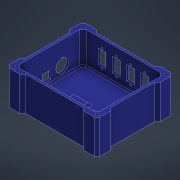
# Autodesk Inventor part: Case
Saved by Autodesk Inventor 2021.3 (Build 253353000, 353)
## iProperties
Created: 2020-02-03
Part Number: Case
Material: Generic
Document SubType Name: Modeling
Designer: Alex
Density: 1 g/cm^3
Appearance: Default
Author: Alex
Autodesk Inventor part; units mm, degrees
ref_plane "YZ Plane" through (0, 0, 0) normal (1, 0, 0) x (0, 1, 0)
ref_plane "XZ Plane" through (0, 0, 0) normal (0, 1, 0) x (-1, 0, 0)
ref_plane "XY Plane" through (0, 0, 0) normal (0, 0, 1) x (1, 0, 0)
sketch "Sketch1" plane through (0, 0, 0) normal (0, 1, 0) x (-1, 0, 0)
  line L0 (-60, 50) -> (-41, 50) construction
  line L1 (60, 50) -> (60, 31) construction
  line L2 (60, -50) -> (41, -50) construction
  line L3 (-60, -50) -> (-60, -31) construction
  line L4 (-60, 50) -> (60, -50) construction
  line L5 (60, 50) -> (-60, -50) construction
  line L6 (41, -50) -> (45, -54)
  line L7 (45, -54) -> (60, -54)
  line L8 (60, -54) -> (64, -50)
  line L9 (64, -50) -> (64, -35)
  line L10 (64, -35) -> (60, -31)
  line L11 (-41, -50) -> (-45, -54)
  line L12 (-45, -54) -> (-60, -54)
  line L13 (-60, -54) -> (-64, -50)
  line L14 (-64, -50) -> (-64, -35)
  line L15 (-64, -35) -> (-60, -31)
  line L16 (-60, 31) -> (-64, 35)
  line L17 (-64, 35) -> (-64, 50)
  line L18 (-64, 50) -> (-60, 54)
  line L19 (-60, 54) -> (-45, 54)
  line L20 (-45, 54) -> (-41, 50)
  line L21 (41, 50) -> (45, 54)
  line L22 (45, 54) -> (60, 54)
  line L23 (60, 54) -> (64, 50)
  line L24 (64, 50) -> (64, 35)
  line L25 (64, 35) -> (60, 31)
  line L26 (41, -50) -> (-41, -50)
  line L27 (60, -31) -> (60, -50) construction
  line L28 (60, 31) -> (60, -31)
  line L29 (41, 50) -> (60, 50) construction
  line L30 (-41, 50) -> (41, 50)
  line L31 (-60, 31) -> (-60, 50) construction
  line L32 (-41, -50) -> (-60, -50) construction
  line L33 (-60, -31) -> (-60, 31)
  point P0 (0, 0)
  point P1 (0, 0)
  point P2 (0, 0)
  dimension "d4" = 120
  dimension "d5" = 100
  dimension "d6" = 45
  dimension "d7" = 15
  dimension "d8" = 4
  dimension "d9" = 4
  dimension "d12" = 45
  dimension "d13" = 4
  constraints: 68 end point, 21 parallel, 16 perpendicular, 7 equal length, 6 collinear, 6 vertical alignment, 5 horizontal, 3 horizontal alignment, 3 midpoint, 1 coincident, 1 point on line
  measures "d4" distance of L2.start L3.start
  measures "d5" distance of L1.start L2.start
  measures "d6" angle of L6 L2
  measures "d7" distance of L6.end L7.end
  measures "d8" distance between parallel lines of L7 L2
  measures "d9" horizontal distance of L7.end L8.end
  measures "d12" angle of L2 L11
  measures "d13" distance between parallel lines of L14 L3
extrude "Extrusion2" add sketch "Sketch1" along normal blind 3
sketch "Sketch2" plane through (0, 3, 0) normal (0, 1, 0) x (1, 0, 0)
  line L0 (-64, 50) -> (-64, 35) projected
  line L1 (-64, 35) -> (-60, 31) projected
  line L2 (-60, 31) -> (-60, -31) projected
  line L3 (-60, -31) -> (-64, -35) projected
  line L4 (-64, -35) -> (-64, -50) projected
  line L5 (-64, -50) -> (-60, -54) projected
  line L6 (-60, -54) -> (-45, -54) projected
  line L7 (-45, -54) -> (-41, -50) projected
  line L8 (-41, -50) -> (41, -50) projected
  line L9 (41, -50) -> (45, -54) projected
  line L10 (45, -54) -> (60, -54) projected
  line L11 (60, -54) -> (64, -50) projected
  line L12 (64, -50) -> (64, -35) projected
  line L13 (64, -35) -> (60, -31) projected
  line L14 (60, -31) -> (60, 31) projected
  line L15 (60, 31) -> (64, 35) projected
  line L16 (64, 35) -> (64, 50) projected
  line L17 (64, 50) -> (60, 54) projected
  line L18 (60, 54) -> (45, 54) projected
  line L19 (45, 54) -> (41, 50) projected
  line L20 (41, 50) -> (-41, 50) projected
  line L21 (-41, 50) -> (-45, 54) projected
  line L22 (-45, 54) -> (-60, 54) projected
  line L23 (-60, 54) -> (-64, 50) projected
  line L24 (-42.2426, 47) -> (42.2426, 47)
  line L25 (42.2426, 47) -> (46.2426, 51) construction
  line L26 (46.2426, 51) -> (58.7574, 51) construction
  line L27 (58.7574, 51) -> (61, 48.7574) construction
  line L28 (61, 48.7574) -> (61, 36.2426) construction
  line L29 (61, 36.2426) -> (57, 32.2426) construction
  line L30 (57, 32.2426) -> (57, -32.2426)
  line L31 (57, -32.2426) -> (61, -36.2426) construction
  line L32 (61, -36.2426) -> (61, -48.7574) construction
  line L33 (61, -48.7574) -> (58.7574, -51) construction
  line L34 (58.7574, -51) -> (46.2426, -51) construction
  line L35 (46.2426, -51) -> (42.2426, -47) construction
  line L36 (42.2426, -47) -> (-42.2426, -47)
  line L37 (-42.2426, -47) -> (-46.2426, -51) construction
  line L38 (-46.2426, -51) -> (-58.7574, -51) construction
  line L39 (-58.7574, -51) -> (-61, -48.7574) construction
  line L40 (-61, -48.7574) -> (-61, -36.2426) construction
  line L41 (-61, -36.2426) -> (-57, -32.2426) construction
  line L42 (-57, -32.2426) -> (-57, 32.2426)
  line L43 (-57, 32.2426) -> (-61, 36.2426) construction
  line L44 (-61, 36.2426) -> (-61, 48.7574) construction
  line L45 (-61, 48.7574) -> (-58.7574, 51) construction
  line L46 (-58.7574, 51) -> (-46.2426, 51) construction
  line L47 (-46.2426, 51) -> (-42.2426, 47) construction
  line L48 (-42.2426, 47) -> (-52.2426, 47)
  line L49 (-52.2426, 47) -> (-57, 42.2426)
  line L50 (-57, 42.2426) -> (-57, 32.2426)
  line L51 (-57, -32.2426) -> (-57, -42.2426)
  line L52 (-57, -42.2426) -> (-52.2426, -47)
  line L53 (-52.2426, -47) -> (-42.2426, -47)
  line L54 (42.2426, -47) -> (52.2426, -47)
  line L55 (52.2426, -47) -> (57, -42.2426)
  line L56 (57, -42.2426) -> (57, -32.2426)
  line L57 (57, 32.2426) -> (57, 42.2426)
  line L58 (57, 42.2426) -> (52.2426, 47)
  line L59 (52.2426, 47) -> (42.2426, 47)
  point P0 (0, 0)
  dimension "d16" = 3
  dimension "d17" = 10
  constraints: 72 end point, 7 equal length, 4 perpendicular, 2 point on line, 1 horizontal, 1 vertical, 23 other
  measures "d16" distance between parallel lines of L20 L24
  measures "d17" distance of L24.start L48.end
extrude "Extrusion3" add sketch "Sketch2" along normal blind 45
sketch "Sketch4" plane through (0, 3, 0) normal (0, 1, 0) x (1, 0, 0)
  line L0 (45, 54) -> (41, 50) construction
  line L1 (41, 50) -> (-41, 50) construction
  line L2 (-41, 50) -> (-45, 54) construction
  line L3 (-45, 54) -> (-60, 54) construction
  line L4 (-60, 54) -> (-64, 50) construction
  line L5 (-64, 50) -> (-64, 35) construction
  line L6 (-64, 35) -> (-60, 31) construction
  line L7 (-60, 31) -> (-60, -31) construction
  line L8 (-60, -31) -> (-64, -35) construction
  line L9 (-64, -35) -> (-64, -50) construction
  line L10 (-64, -50) -> (-60, -54) construction
  line L11 (-60, -54) -> (-45, -54) construction
  line L12 (-45, -54) -> (-41, -50) construction
  line L13 (-41, -50) -> (41, -50) construction
  line L14 (41, -50) -> (45, -54) construction
  line L15 (45, -54) -> (60, -54) construction
  line L16 (60, -54) -> (64, -50) construction
  line L17 (64, -50) -> (64, -35) construction
  line L18 (64, -35) -> (60, -31) construction
  line L19 (60, -31) -> (60, 31) construction
  line L20 (60, 31) -> (64, 35) construction
  line L21 (64, 35) -> (64, 50) construction
  line L22 (64, 50) -> (60, 54) construction
  line L23 (60, 54) -> (45, 54) construction
  line L24 (-52.2426, 47) -> (52.2426, 47) construction
  line L25 (52.2426, 47) -> (57, 42.2426) construction
  line L26 (57, 42.2426) -> (57, -42.2426) construction
  line L27 (57, -42.2426) -> (52.2426, -47) construction
  line L28 (52.2426, -47) -> (-52.2426, -47) construction
  line L29 (-52.2426, -47) -> (-57, -42.2426) construction
  line L30 (-57, -42.2426) -> (-57, 42.2426) construction
  line L31 (-57, 42.2426) -> (-52.2426, 47) construction
  line L32 (-52.2426, 47) -> (-57, 42.2426) construction
  line L33 (-57, 42.2426) -> (-57, -42.2426) construction
  line L34 (-57, -42.2426) -> (-52.2426, -47) construction
  line L35 (-52.2426, -47) -> (52.2426, -47) construction
  line L36 (52.2426, -47) -> (57, -42.2426) construction
  line L37 (57, -42.2426) -> (57, 42.2426) construction
  line L38 (57, 42.2426) -> (52.2426, 47) construction
  line L39 (52.2426, 47) -> (-52.2426, 47) construction
  line L40 (-54, 11.34) -> (47.6, 11.34) construction
  line L41 (47.6, 11.34) -> (47.6, -42) construction
  line L42 (47.6, -42) -> (-54, -42) construction
  line L43 (-54, -42) -> (-54, 11.34) construction
  line L44 (9.6, -4) -> (14.6, -4)
  line L45 (14.6, -4) -> (14.6, -9)
  line L46 (14.6, -9) -> (9.6, -9)
  line L47 (9.6, -9) -> (9.6, -4)
  line L48 (9.6, -4) -> (14.6, -9) construction
  line L49 (14.6, -4) -> (9.6, -9) construction
  line L50 (45.02, -42) -> (40.02, -42)
  line L51 (40.02, -42) -> (40.02, -37)
  line L52 (40.02, -37) -> (45.02, -37)
  line L53 (45.02, -37) -> (45.02, -42)
  line L54 (45.02, -42) -> (40.02, -37) construction
  line L55 (40.02, -42) -> (45.02, -37) construction
  line L56 (-24, 1.34) -> (-4, 1.34)
  line L57 (-4, 1.34) -> (-4, -32)
  line L58 (-4, -32) -> (-24, -32)
  line L59 (-24, -32) -> (-24, 1.34)
  line L60 (21, 1.34) -> (31, 1.34)
  line L61 (31, 1.34) -> (31, -32)
  line L62 (31, -32) -> (21, -32)
  line L63 (21, -32) -> (21, 1.34)
  point P0 (-40, -39.5)
  point P1 (-38.7, 8.7)
  point P2 (12.1, -34.4)
  point P3 (12.1, -6.5)
  point P4 (36.2, 8.7)
  point P5 (42.52, -39.5)
  dimension "d20" = 53.34
  dimension "d21" = 101.6
  dimension "d23" = 5
  dimension "d24" = 3
  dimension "d25" = 14
  dimension "d26" = 1.3
  dimension "d27" = 50.8
  dimension "d29" = 2.5
  dimension "d30" = 5.1
  dimension "d31" = 27.9
  dimension "d32" = 15.2
  dimension "d33" = 24.1
  dimension "d34" = 96.52
  dimension "d35" = 30
  dimension "d36" = 50
  dimension "d37" = 10
  dimension "d38" = 10
  dimension "d39" = 75
  dimension "d40" = 85
  dimension "d41" = 5
  constraints: 48 end point, 10 parallel, 5 horizontal, 5 perpendicular, 4 midpoint, 3 equal length, 2 collinear, 2 horizontal alignment, 1 vertical alignment
  measures "d20" distance of L40.end L41.end
  measures "d21" distance of L40.start L40.end
  measures "d23" distance between parallel lines of L42 L28
  measures "d24" distance between parallel lines of L30 L43
  measures "d25" distance from line of point (-40, -39.5) L43
  measures "d26" horizontal distance of point (-38.7, 8.7) point (-40, -39.5)
  measures "d27" horizontal distance of point (12.1, -6.5) point (-38.7, 8.7)
  measures "d29" distance from line of point (42.52, -39.5) L42
  measures "d30" vertical distance of point (12.1, -34.4) point (-40, -39.5)
  measures "d31" distance of point (12.1, -6.5) point (12.1, -34.4)
  measures "d32" vertical distance of point (36.2, 8.7) point (12.1, -6.5)
  measures "d33" horizontal distance of point (36.2, 8.7) point (12.1, -6.5)
  measures "d34" distance from line of point (42.52, -39.5) L43
  measures "d35" distance between parallel lines of L59 L43
  measures "d36" distance between parallel lines of L57 L43
  measures "d37" distance between parallel lines of L56 L40
  measures "d38" distance between parallel lines of L58 L42
  measures "d39" distance between parallel lines of L63 L43
  measures "d40" distance between parallel lines of L61 L43
  measures "d41" distance of L45.end L46.end
extrude "Extrusion4" add sketch "Sketch4" along normal blind 3
chamfer "Chamfer1" distance 3 angle 45 16 edges at (-14, 3, 32) (-4, 3, 15.33) (21, 3, 15.33) (-24, 3, 15.33) (26, 3, 32) (40.02, 3, 39.5) (42.52, 3, 37) (45.02, 3, 39.5) (42.52, 3, 42) (9.6, 3, 6.5) (12.1, 3, 9) (14.6, 3, 6.5) (12.1, 3, 4) (26, 3, -1.34) (-14, 3, -1.34) (31, 3, 15.33)
sketch "Sketch5" plane through (0, 6, 0) normal (0, 1, 0) x (1, 0, 0)
  line L0 (14.6, -9) -> (14.6, -4) construction
  line L1 (14.6, -4) -> (9.6, -4) construction
  line L2 (9.6, -4) -> (9.6, -9) construction
  line L3 (9.6, -9) -> (14.6, -9) construction
  line L4 (40.02, -42) -> (45.02, -42) construction
  line L5 (45.02, -42) -> (45.02, -37) construction
  line L6 (45.02, -37) -> (40.02, -37) construction
  line L7 (40.02, -37) -> (40.02, -42) construction
  point P0 (0, 0)
  point P1 (12.1, -6.5)
  point P2 (42.52, -39.5)
  point P3 (14.6, -6.5)
  point P4 (45.02, -39.5)
  point P5 (12.1, -4)
  point P6 (42.52, -37)
  constraints: 4 midpoint, 2 horizontal alignment, 2 vertical alignment
hole "Hole1" at (12.1, 6, 6.5) at (42.52, 6, 39.5) direction (0, -1, 0) diameter 4 depth 5
sketch "Sketch6" plane through (-57, 3, 42.2426) normal (1, 0, 0) x (0, 0, -1)
  line L0 (46.5826, 0) -> (7.2426, 0) construction
  line L1 (7.2426, 0) -> (46.5826, 0) construction
  line L2 (7.2426, 0) -> (46.5826, 0) construction
  line L3 (46.5826, 0) -> (7.2426, 0) construction
  line L4 (-2.7574, 0) -> (8.2426, 0) construction
  line L5 (-4.7574, 0) -> (0, 0) construction
  line L6 (0, 0) -> (84.4853, 0) construction
  line L7 (84.4853, 0) -> (89.2426, 0) construction
  line L8 (89.2426, 0) -> (84.4853, 0) construction
  line L9 (84.4853, 0) -> (0, 0) construction
  line L10 (0, 0) -> (-4.7574, 0) construction
  line L11 (8.2426, 0) -> (-2.7574, 0) construction
  line L12 (41.2426, 0) -> (30.2426, 0) construction
  line L13 (30.2426, 0) -> (41.2426, 0) construction
  line L14 (0.2426, 0) -> (53.5826, 0) construction
  line L15 (43.5826, 3) -> (10.2426, 3) construction
  line L16 (10.2426, 3) -> (43.5826, 3) construction
  line L17 (43.5826, 3) -> (46.5826, 0) construction
  line L18 (46.5826, 0) -> (43.5826, 3) construction
  line L19 (10.2426, 3) -> (7.2426, 0) construction
  line L20 (10.2426, 3) -> (7.2426, 0) construction
  line L21 (84.4853, 0) -> (0, 0) construction
  line L22 (84.4853, 0) -> (84.4853, 45) construction
  line L23 (0, 45) -> (84.4853, 45) construction
  line L24 (0, 0) -> (0, 45) construction
  line L25 (31.8326, 16.2) -> (44.3326, 16.2)
  line L26 (44.3326, 16.2) -> (44.3326, 4.7)
  line L27 (44.3326, 4.7) -> (31.8326, 4.7)
  line L28 (31.8326, 4.7) -> (31.8326, 16.2)
  point P0 (42.2426, -3)
  dimension "d55" = 11.5
  dimension "d56" = 12.5
  dimension "d57" = 1.7
  dimension "d58" = 9.25
  constraints: 8 end point, 2 parallel, 1 horizontal, 1 perpendicular, 1 other
  measures "d55" distance between parallel lines of L25 L27
  measures "d56" distance between parallel lines of L26 L28
  measures "d57" distance between parallel lines of L27 L15
  measures "d58" distance from line of point (53.583, 0) L26
extrude "Extrusion5" cut sketch "Sketch6" against normal blind 10
sketch "Sketch7" plane through (0, 48, 0) normal (0, 1, 0) x (1, 0, 0)
  line L0 (41, -50) -> (45, -54) construction
  line L1 (45, -54) -> (60, -54) construction
  line L2 (60, -54) -> (64, -50) construction
  line L3 (64, -50) -> (64, -35) construction
  line L4 (64, -35) -> (60, -31) construction
  line L5 (60, -31) -> (60, 31) construction
  line L6 (60, 31) -> (64, 35) construction
  line L7 (64, 35) -> (64, 50) construction
  line L8 (64, 50) -> (60, 54) construction
  line L9 (60, 54) -> (45, 54) construction
  line L10 (45, 54) -> (41, 50) construction
  line L11 (41, 50) -> (-41, 50) construction
  line L12 (-41, 50) -> (-45, 54) construction
  line L13 (-45, 54) -> (-60, 54) construction
  line L14 (-60, 54) -> (-64, 50) construction
  line L15 (-64, 50) -> (-64, 35) construction
  line L16 (-64, 35) -> (-60, 31) construction
  line L17 (-60, 31) -> (-60, -31) construction
  line L18 (-60, -31) -> (-64, -35) construction
  line L19 (-64, -35) -> (-64, -50) construction
  line L20 (-64, -50) -> (-60, -54) construction
  line L21 (-60, -54) -> (-45, -54) construction
  line L22 (-45, -54) -> (-41, -50) construction
  line L23 (-41, -50) -> (41, -50) construction
  line L24 (52.2426, -47) -> (-52.2426, -47) construction
  line L25 (-52.2426, -47) -> (-57, -42.2426) construction
  line L26 (-57, -42.2426) -> (-57, 42.2426) construction
  line L27 (-57, 42.2426) -> (-52.2426, 47) construction
  line L28 (-52.2426, 47) -> (52.2426, 47) construction
  line L29 (52.2426, 47) -> (57, 42.2426) construction
  line L30 (57, 42.2426) -> (57, -42.2426) construction
  line L31 (57, -42.2426) -> (52.2426, -47) construction
  line L32 (-64, -35) -> (-64, -50) construction
  line L33 (-57, -42.2426) -> (-52.2426, -47) construction
  line L34 (-64, -50) -> (-52.2426, -47) construction
  line L35 (-60, -54) -> (-45, -54) construction
  line L36 (-57, -42.2426) -> (-57, 42.2426) construction
  line L37 (-60, -54) -> (-57, -42.2426) construction
  line L38 (-57, 0) -> (57, 0) construction
  line L39 (57, -42.2426) -> (57, 42.2426) projected
  line L40 (-52.2426, -47) -> (52.2426, -47) projected
  line L41 (0, -50) -> (0, 50) construction
  line L42 (41, 50) -> (-41, 50) projected
  point P0 (0, 0)
  point P1 (-58.6297, -48.6297)
  point P2 (37.02, -47)
  point P3 (58.6297, -48.6297)
  point P4 (-58.6297, 48.6297)
  point P5 (58.6297, 48.6297)
  constraints: 8 end point, 4 midpoint, 3 symmetric about line, 2 point on line
hole "Hole2" at (-58.6297, 48, 48.6297) at (58.6297, 48, 48.6297) at (58.6297, 48, -48.6297) at (-58.6297, 48, -48.6297) direction (0, -1, 0) diameter 4 depth 5
sketch "Sketch8" plane through (-60, 0, -31) normal (-1, 0, 0) x (0, 0, 1)
  line L0 (28.91, 7.7) -> (28.91, 19.2) construction
  line L1 (28.91, 19.2) -> (41.41, 19.2) construction
  line L2 (41.41, 19.2) -> (41.41, 7.7) construction
  line L3 (41.41, 7.7) -> (28.91, 7.7) construction
  line L4 (0, 0) -> (62, 0) construction
  line L5 (62, 0) -> (62, 48) construction
  line L6 (0, 48) -> (62, 48) construction
  line L7 (0, 0) -> (0, 48) construction
  line L8 (28.91, 19.2) -> (28.91, 7.7) construction
  line L9 (28.91, 7.7) -> (41.41, 7.7) construction
  line L10 (41.41, 7.7) -> (41.41, 19.2) construction
  line L11 (41.41, 19.2) -> (28.91, 19.2) construction
  line L12 (-11.2426, 3) -> (73.2426, 3) construction
  line L13 (-11.2426, 3) -> (-11.2426, 48) construction
  line L14 (73.2426, 48) -> (-11.2426, 48) construction
  line L15 (73.2426, 3) -> (73.2426, 48) construction
  arc A0 (11.5, 24.8741) -> (14.5, 24.8741) centre (13, 16) ccw
  circle A1 centre (13, 16) radius 10 construction
  line L16 (11.5, 25.8869) -> (11.5, 6.1131) construction
  line L17 (14.5, 25.8869) -> (14.5, 6.1131) construction
  line L18 (11.5, 16) -> (13, 16) construction
  line L19 (13, 16) -> (14.5, 16) construction
  line L20 (11.5, 24.8741) -> (11.5, 25.8869)
  line L21 (14.5, 24.8741) -> (14.5, 25.8869)
  arc A2 (14.5, 24.8741) -> (11.5, 24.8741) centre (13, 16) ccw construction
  arc A3 (14.5, 25.8869) -> (11.5, 25.8869) centre (13, 16) ccw
  point P0 (31, 0)
  dimension "d68" = 18
  dimension "d69" = 20
  dimension "d70" = 3
  dimension "d71" = 13
  dimension "d72" = 13
  constraints: 12 end point, 10 point on circle, 4 centre point, 3 collinear, 2 coincident, 2 midpoint, 2 point on line, 2 vertical, 1 horizontal
  measures "d68" diameter of A0
  measures "d69" diameter of A1
  measures "d70" distance between parallel lines of L16 L17
  measures "d71" distance from line of L12 A0.centre
  measures "d72" distance from line of L7 A0.centre
extrude "Extrusion6" cut sketch "Sketch8" against normal blind 10
sketch "Sketch10" plane through (41, 0, -50) normal (0, 0, -1) x (-1, 0, 0)
  line L0 (5.5, 34) -> (16.5, 34)
  line L1 (16.5, 34) -> (16.5, 14)
  line L2 (16.5, 14) -> (5.5, 14)
  line L3 (5.5, 14) -> (5.5, 34)
  line L4 (4.5, 39.5) -> (17.5, 39.5) construction
  line L5 (17.5, 39.5) -> (17.5, 8.5) construction
  line L6 (17.5, 8.5) -> (4.5, 8.5) construction
  line L7 (4.5, 8.5) -> (4.5, 39.5) construction
  line L8 (0, 0) -> (82, 0) construction
  line L9 (82, 0) -> (82, 48) construction
  line L10 (0, 48) -> (82, 48) construction
  line L11 (0, 0) -> (0, 48) construction
  line L12 (24.5, 39.5) -> (37.5, 39.5) construction
  line L13 (25.5, 34) -> (36.5, 34)
  line L14 (36.5, 34) -> (36.5, 14)
  line L15 (36.5, 14) -> (25.5, 14)
  line L16 (25.5, 14) -> (25.5, 34)
  line L17 (37.5, 39.5) -> (37.5, 8.5) construction
  line L18 (24.5, 8.5) -> (24.5, 39.5) construction
  line L19 (37.5, 8.5) -> (24.5, 8.5) construction
  line L20 (44.5, 39.5) -> (57.5, 39.5) construction
  line L21 (45.5, 34) -> (56.5, 34)
  line L22 (56.5, 34) -> (56.5, 14)
  line L23 (56.5, 14) -> (45.5, 14)
  line L24 (45.5, 14) -> (45.5, 34)
  line L25 (57.5, 39.5) -> (57.5, 8.5) construction
  line L26 (44.5, 8.5) -> (44.5, 39.5) construction
  line L27 (57.5, 8.5) -> (44.5, 8.5) construction
  line L28 (64.5, 39.5) -> (77.5, 39.5) construction
  line L29 (65.5, 34) -> (76.5, 34)
  line L30 (76.5, 34) -> (76.5, 14)
  line L31 (76.5, 14) -> (65.5, 14)
  line L32 (65.5, 14) -> (65.5, 34)
  line L33 (77.5, 39.5) -> (77.5, 8.5) construction
  line L34 (64.5, 8.5) -> (64.5, 39.5) construction
  line L35 (77.5, 8.5) -> (64.5, 8.5) construction
  line L36 (0, 48) -> (82, 48) construction
  line L37 (41, 48) -> (41, 0) construction
  point P0 (11, 39.5)
  point P1 (11, 34)
  point P2 (5.5, 24)
  point P3 (4.5, 24)
  point P4 (31, 39.5)
  point P5 (31, 34)
  point P6 (25.5, 24)
  point P7 (24.5, 24)
  point P8 (51, 39.5)
  point P9 (51, 34)
  point P10 (45.5, 24)
  point P11 (44.5, 24)
  point P12 (71, 39.5)
  point P13 (71, 34)
  point P14 (65.5, 24)
  point P15 (64.5, 24)
  point P16 (0, 24)
  dimension "d75" = 13
  dimension "d76" = 11
  dimension "d77" = 31
  dimension "d78" = 20
  dimension "d81" = 20
  constraints: 66 end point, 6 midpoint, 4 parallel, 3 horizontal, 2 horizontal alignment, 2 perpendicular, 1 collinear, 1 vertical, 1 vertical alignment, 60 other
  measures "d75" distance of L4.start L4.end
  measures "d76" distance of L0.start L0.end
  measures "d77" distance of L4.end L5.end
  measures "d78" distance of L0.end L1.end
  measures "d81" distance of L0.end L13.end
extrude "Extrusion7" cut sketch "Sketch10" against normal blind 5
sketch "Sketch11" plane through (41, 0, -50) normal (0, 0, -1) x (-1, 0, 0)
  line L0 (56.5, 34) -> (56.5, 14) construction
  line L1 (56.5, 14) -> (45.5, 14) construction
  line L2 (45.5, 14) -> (45.5, 34) construction
  line L3 (45.5, 34) -> (56.5, 34) construction
  line L4 (36.5, 34) -> (36.5, 14) construction
  line L5 (36.5, 14) -> (25.5, 14) construction
  line L6 (25.5, 14) -> (25.5, 34) construction
  line L7 (25.5, 34) -> (36.5, 34) construction
  line L8 (76.5, 34) -> (76.5, 14) construction
  line L9 (76.5, 14) -> (65.5, 14) construction
  line L10 (65.5, 14) -> (65.5, 34) construction
  line L11 (65.5, 34) -> (76.5, 34) construction
  line L12 (16.5, 34) -> (16.5, 14) construction
  line L13 (16.5, 14) -> (5.5, 14) construction
  line L14 (5.5, 14) -> (5.5, 34) construction
  line L15 (5.5, 34) -> (16.5, 34) construction
  line L16 (0, 0) -> (82, 0) construction
  line L17 (82, 0) -> (82, 48) construction
  line L18 (0, 48) -> (82, 48) construction
  line L19 (0, 0) -> (0, 48) construction
  line L20 (11, 36.5) -> (11, 11.5) construction
  point P0 (41, 0)
  point P1 (5.5, 24)
  point P2 (11, 24)
  point P3 (11, 34)
  point P4 (31, 36.5)
  point P5 (31, 11.5)
  point P6 (51, 36.5)
  point P7 (51, 11.5)
  point P8 (71, 36.5)
  point P9 (71, 11.5)
  dimension "d88" = 25
  dimension "d91" = 20
  constraints: 3 midpoint, 2 end point, 1 horizontal, 1 horizontal alignment, 1 point on line, 1 vertical, 6 other
  measures "d88" distance of L20.end L20.start
  measures "d91" distance of L20.start point (31, 36.5)
hole "Hole3" at (30, 36.5, -50) at (30, 11.5, -50) at (10, 36.5, -50) at (10, 11.5, -50) at (-10, 36.5, -50) at (-10, 11.5, -50) at (-30, 36.5, -50) at (-30, 11.5, -50) direction (0, 0, 1) diameter 2.9 depth 3 clearance for "Socket Head Cap Screw ISO 4762" size "M2.5" standard "ISO"
chamfer "Chamfer2" distance 2 angle 45 8 edges at (57, 3, 0) (0, 3, -47) (54.6213, 3, -44.6213) (-54.6213, 3, -44.6213) (-57, 3, 0) (0, 3, 47) (-54.6213, 3, 44.6213) (54.6213, 3, 44.6213)
equation "\"d9\" = d8"
equation "\"d13\" = d9"
body "Solid2"
